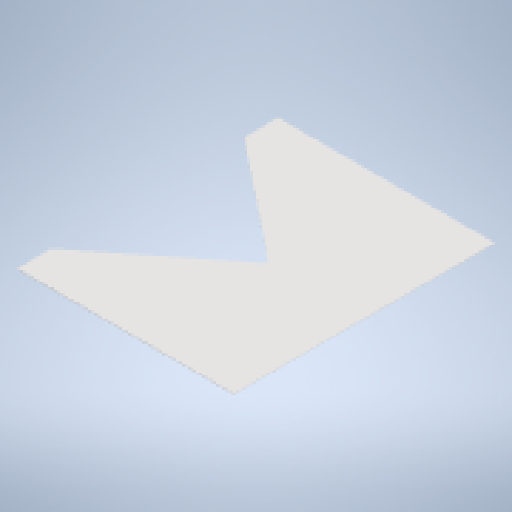
# Autodesk Inventor part: BSH 033 board cone 3
Saved by Autodesk Inventor 2025 (Build 290162010, 162A)
## iProperties
Created: 2024-07-23
Part Number: BSH 033 board cone 3
Material: 09g2s
Document SubType Name: Sheet Metal
Designer: admin
Density: 7.85 g/cm^3
Flat Pattern Width: 134.5 cm
Flat Pattern Length: 162 cm
Flat Pattern Area: 21789 cm^2
Sheet Metal Rule: AISI304 3mm Die 32
Sheet Metal Width: 1345,000 mm
Sheet Metal Length: 1620,000 mm
Sheet Metal Area: 2178900,000 mm^2
Appearance: Default
Mass: 40581.4 g
Surface Area: 34651.2 cm^2
Volume: 5169.6 cm^3
Author: admin
Autodesk Inventor part; units mm, degrees
ref_plane "YZ Plane" through (0, 0, 0) normal (1, 0, 0) x (0, 1, 0)
ref_plane "XZ Plane" through (0, 0, 0) normal (0, 1, 0) x (-1, 0, 0)
ref_plane "XY Plane" through (0, 0, 0) normal (0, 0, 1) x (1, 0, 0)
sketch "Sketch1" plane through (0, 0, 0) normal (0, 0, 1) x (1, 0, 0)
  line L0 (0, -810) -> (1345, -810)
  line L1 (1345, -810) -> (1345, 810)
  line L2 (1345, 810) -> (0, 810)
  line L3 (0, 810) -> (0, -810)
  point P0 (0, 0)
  point P1 (0, 0)
  dimension "d0" = 1345
  dimension "d1" = 1620
  measures "d0" distance of L2.end L1.end
  measures "d1" distance of L1.end L0.end
extrude "Plate1" add sketch "Sketch1" along normal blind 3
sketch "Sketch5" plane through (0, 0, 0) normal (0, 0, -1) x (-1, 0, 0)
  line L0 (0, -810) -> (-1345, -810) construction
  line L1 (0, 810) -> (0, -810) projected
  line L2 (-1345, 810) -> (0, 810) construction
  line L3 (-1345, -810) -> (-1345, 810) construction
  line L4 (0, -600) -> (-750, 0)
  line L5 (-750, 0) -> (0, 600)
  line L6 (12.3081, -1975.0573) -> (-487.6919, -1975.0573)
  line L7 (-487.6919, -1975.0573) -> (-487.6919, -2425.2593)
  line L8 (-487.6919, -2425.2593) -> (12.3081, -1975.0573)
  point P0 (0, 0)
  point P1 (0, 0)
  dimension "d26" = 500
  dimension "d27" = 48
  dimension "d28" = 672.8164
  dimension "d29" = 750
  dimension "d30" = 1200
  constraints: 10 end point, 2 point on line, 1 equal length, 1 horizontal, 1 horizontal alignment, 1 midpoint, 1 perpendicular
  measures "d26" distance of L6.start L6.end
  measures "d27" angle of L8 L7
  measures "d28" distance of L7.end L6.start
  measures "d29" distance from line of L1 L4.end
  measures "d30" distance of L5.end L4.start
extrude "Cut1" cut sketch "Sketch5" against normal blind 3 contours L1 L4 L5
equation "\"d31\" = Thickness"
equation "\"d2\" = Thickness"
equation "\"BendReliefWidth\" = Thickness"
equation "\"BendReliefDepth\" = 0.5 * Thickness"
equation "\"CornerReliefSize\" = 4 * Thickness"
equation "\"MinimumRemnant\" = 2 * Thickness"
equation "\"TransitionRadius\" = BendRadius"
equation "\"JacobiRadiusSize\" = BendRadius"
equation "\"GapSize\" = Thickness"
equation "\"Thickness\" = 3"
equation "\"BendRadius\" = 5"
body "Solid1"
